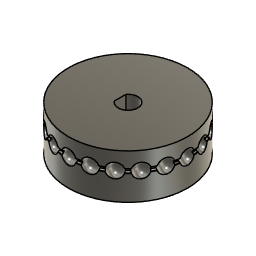
chain_sprocket (Autodesk Fusion 360 design; units mm, degrees)
Autodesk Fusion 360 part; units mm, degrees
sketch "Sketch1" plane through (0, 0, 0) normal (0, 0, 1) x (1, 0, 0)
  circle A0 centre (0, 0) radius 18.7328
  line L0 (2.4, 1.8) -> (2.4, -1.8) construction
  arc A1 (2.4, 1.8) -> (2.4, -1.8) centre (0, 0) ccw construction
  line L1 (2.4875, 1.8289) -> (2.4875, -1.8289)
  arc A2 (2.4875, 1.8289) -> (2.4875, -1.8289) centre (0, 0) ccw
  dimension "d1" = 37.4656
  dimension "d2" = 6
  dimension "d3" = 2.4
  dimension "d4" = 0.0875
  constraint coincident A0.centre A1.centre
  constraint concentric A0 A1
  constraint vertical L0
  measures "d1" diameter of A0
  measures "d2" diameter of A1
  measures "d3" distance of A0.centre L0
extrude "Extrude1" add sketch "Sketch1" along normal blind 12
sketch "Sketch2" plane through (0, 0, 12) normal (0, 0, 1) x (1, 0, 0)
  arc A0 (2.4875, 1.8289) -> (2.4875, -1.8289) centre (0, 0) ccw
  line L0 (2.4875, 1.8289) -> (2.4875, -1.8289)
  circle A1 centre (0, 0) radius 18.7328
  circle A2 centre (0, 0) radius 1.5875
  dimension "d7" = 3.175
  constraint concentric A0 A2
  measures "d7" diameter of A2
extrude "Extrude2" add sketch "Sketch2" along normal blind 2 contours A0 L0 | A1
sketch "Sketch3" plane through (0, 0, 0) normal (1, 0, 0) x (0, 0, -1)
  circle A0 through (-14, 18.7328, 0) (-14, -9.3664, 16.2231) (-14, -9.3664, -16.2231)
  line L0 (0, 0) -> (-14, 0)
  line L1 (-3.35, 6.1343) -> (-3.35, -3.5456) construction
  line L2 (-7.65, 18.7328) -> (-7.65, -2.9906) construction
  line L3 (0, 18.7328) -> (0, -18.7328)
  line L4 (0, 18.7328) -> (-4.8476, 18.7328) construction
  line L5 (-5.5, 0) -> (-5.5, 18.7328) construction
  line L6 (-5.5, 0) -> (-5.5, 18.3028) construction
  circle A1 centre (-5.5, 18.3028) radius 2.15 construction
  circle A2 centre (-5.5, 18.4298) radius 2.15 construction
  circle A3 centre (-5.5, 18.4298) radius 2.277
  circle A4 centre (-5.5, 18.3028) radius 0.3
  line L7 (-3.223, 18.4298) -> (-7.777, 18.4298)
  line L8 (-5.2402, 18.1528) -> (-4.9342, 18.6828)
  line L9 (-5.7598, 18.1528) -> (-6.0658, 18.6828)
  arc A5 (-4.8476, 18.7328) -> (-4.9342, 18.6828) centre (-4.8476, 18.6328) ccw
  line L10 (-7.65, 18.7328) -> (-6.1524, 18.7328) construction
  arc A6 (-6.0658, 18.6828) -> (-6.1524, 18.7328) centre (-6.1524, 18.6328) ccw
  line L11 (-6.1524, 18.7328) -> (-4.8476, 18.7328)
  dimension "d11" = 3.35
  dimension "d12" = 6.35
  dimension "d28" = 18.3028
  dimension "d29" = 4.3
  dimension "d30" = 4.3
  dimension "d31" = 0.303
  dimension "d32" = 0.127
  dimension "d33" = 0.6
  dimension "d37" = 30
  dimension "d38" = 0.1
  dimension "d39" = 0.1
  constraint coincident L0.start origin
  constraint vertical L1
  constraint vertical L2
  constraint coincident L3.start L4.start
  constraint perpendicular L3 L4
  constraint coincident L4 L5.end
  constraint perpendicular L4 L5
  constraint coincident L0 L5.start
  constraint perpendicular L0 L6
  constraint coincident L6.end A1.centre
  constraint coincident L5 L6.end
  constraint coincident L5 A2.centre
  constraint concentric A1 A4
  constraint tangent L2 A2
  constraint tangent L1 A2
  constraint coincident A4 L8.start
  constraint coincident A4 L9.start
  constraint coincident A3 L7.start
  constraint coincident A3 L7.end
  constraint horizontal L7
  constraint coincident A2.centre L7
  constraint tangent L8 A5
  constraint tangent L4 A5
  constraint horizontal L10
  constraint tangent L9 A6
  constraint tangent L10 A6
  constraint tangent A4 L8
  constraint tangent A4 L9
  constraint equal L8 L9
  constraint horizontal L11
  measures "d11" distance of L1 L3
  measures "d12" distance of L0.end L2
  measures "d28" distance of L5.start L6.end
  measures "d29" diameter of A1
  measures "d30" diameter of A2
  measures "d31" distance of L5.end A2.centre
  measures "d33" diameter of A4
  measures "d37" angle of L5 L8
  measures "d38" radius of A5
  measures "d39" radius of A6
revolve "Revolve2" cut sketch "Sketch3" angle 360 about axis through (0, 18.4298, 3.223) along (0, 0, 1) contours A3 L7 L8 L9 A5 A6 L11 | A4 L7 L8 L9 A5 A6 L11 | A4 L7 picked at (-5.5498, 18.5146)
pattern_circular "C-Pattern2" count 20 over 360 about axis through (0, 0, 1.75) along (0, 0, 1) of "Revolve2"
revolve "Revolve3" cut sketch "Sketch3" angle 360 about axis through (0, 0, 0) along (0, 0, 1) contours A4 L7 L8 | A4 L7 L8 L9 A5 A6 L11 | A4 L7 L9 | A4 L7 | A4 L7
equation "d1 = ( ( 20 * 5.75 / PI ) * 1 mm ) + ( ( 2 * 0.43 ) * 1 mm )"
equation "d3 = 5.4 mm - 3 mm"
equation "d4 = ( 0.175 / 2 ) * 1 mm"
equation "d28 = ( ( 20 * 5.75 / ( 2 * PI ) ) * 1 mm )"
